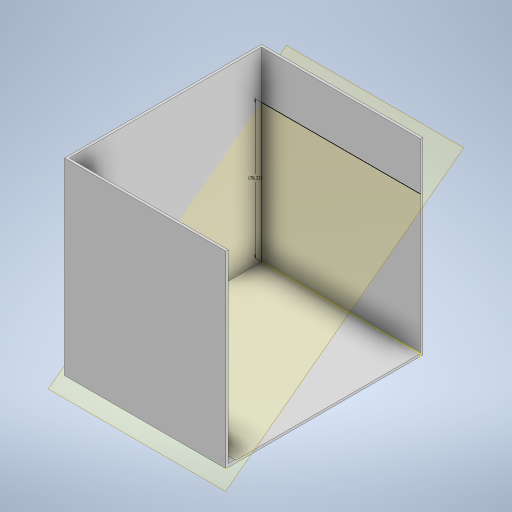
# Autodesk Inventor part: fullsembly
Saved by Autodesk Inventor 2024 (Build 280153000, 153)
## iProperties
Created: 2026-03-21
Part Number: fullsembly
Material: Generic
Document SubType Name: Modeling
Designer: schar
Density: 1 g/cm^3
Appearance: Default
Author: schar
Autodesk Inventor part; units mm, degrees
ref_plane "YZ Plane" through (0, 0, 0) normal (1, 0, 0) x (0, 1, 0)
ref_plane "XZ Plane" through (0, 0, 0) normal (0, 1, 0) x (-1, 0, 0)
ref_plane "XY Plane" through (0, 0, 0) normal (0, 0, 1) x (1, 0, 0)
sketch "Sketch1" plane through (0, 0, 0) normal (0, 1, 0) x (-1, 0, 0)
  line L0 (0, 0) -> (208, 0)
  line L1 (208, 0) -> (208, -254)
  line L2 (208, -254) -> (0, -254)
  line L3 (0, -254) -> (0, 0)
  dimension "d0" = 208
  dimension "d1" = 254
  constraints: 8 end point, 2 parallel, 1 horizontal, 1 perpendicular
  measures "d0" distance of L1.end L2.end
  measures "d1" distance of L0.end L1.end
extrude "Extrusion1" add sketch "Sketch1" along normal blind 3
sketch "Sketch2" plane through (0, 3, 0) normal (0, 1, 0) x (1, 0, 0)
  line L0 (0, 0) -> (0, 254) projected
  line L1 (-208, 254) -> (-208, 0) projected
  line L2 (0, 0) -> (-208, 0)
  line L3 (-208, 0) -> (-208, 3)
  line L4 (-208, 3) -> (0, 3)
  line L5 (0, 3) -> (0, 0)
  line L6 (0, 254) -> (-208, 254)
  line L7 (-208, 254) -> (-208, 251)
  line L8 (-208, 251) -> (0, 251)
  line L9 (0, 251) -> (0, 254)
  line L10 (-208, 3) -> (-205, 3)
  line L11 (-205, 3) -> (-205, 251)
  line L12 (-205, 251) -> (-208, 251)
  line L13 (-208, 251) -> (-208, 3)
  point P0 (-208, 0)
  point P1 (-205, 3)
  dimension "d4" = 3
  dimension "d5" = 3
  dimension "d6" = 3
  constraints: 24 end point, 6 parallel, 3 horizontal, 3 perpendicular, 3 point on line
  measures "d4" distance of L2.end L3.end
  measures "d5" distance of L7.end L6.end
  measures "d6" distance of L12.end L11.end
extrude "Extrusion2" add sketch "Sketch2" along normal blind 240 contours L2 L1 L4 L0 | L8 L1 L6 L0 | L4 L1 L8 L11
sketch "Sketch3" plane through (0, 0, 0) normal (1, 0, 0) x (0, 0, -1)
  point P0 (0, 0)
sketch "Sketch4" plane through (-205, 3, -3) normal (1, 0, 0) x (0, 0, -1)
  line L0 (0, 0) -> (1.4142, 0)
  line L1 (1.4142, 0) -> (1.4142, 1.4142)
  line L2 (1.4142, 1.4142) -> (0, 1.4142)
  line L3 (0, 1.4142) -> (0, 0)
  line L4 (0, 1.4142) -> (1.4142, 0)
  point P0 (-3, -3)
  dimension "d10" = 1.4142
  dimension "d11" = 1.4142
  constraints: 10 end point, 2 parallel, 1 horizontal, 1 perpendicular
  measures "d10" distance of L2.end L1.end
  measures "d11" distance of L1.end L0.end
extrude "Extrusion3" add sketch "Sketch4" along normal up to surface (205 mm away) contours L3 L4 L0
sketch "Sketch5" plane through (-205, 3, -251) normal (1, 0, 0) x (0, 0, -1)
  line L0 (-248, 1.4142) -> (-248, 240) projected
  line L1 (0, 0) -> (-246.5858, 0) projected
  line L2 (-248, 1.4142) -> (-238, 1.4142)
  line L3 (-238, 1.4142) -> (-238, 0)
  line L4 (-238, 0) -> (-248, 0)
  line L5 (-248, 0) -> (-248, 1.4142)
  point P0 (-251, -3)
  dimension "d14" = 10
  constraints: 8 end point, 2 parallel, 1 horizontal, 1 perpendicular, 1 point on line
  measures "d14" distance of L3.end L4.end
extrude "Extrusion4" add sketch "Sketch5" along normal up to surface (205 mm away)
sketch "Sketch6" plane through (0, 0, 0) normal (1, 0, 0) x (0, 0, -1)
  line L0 (13, 4.4142) -> (13, 3) projected
  line L1 (13, 3) -> (11.5858, 4.4142)
  line L2 (3, 4.4142) -> (13, 4.4142) projected
  line L3 (13, 4.4142) -> (11.5858, 4.4142)
  line L4 (13, 4.4142) -> (13, 3)
  point P0 (0, 0)
  dimension "d17" = 2
  constraints: 6 end point, 1 horizontal, 1 perpendicular, 1 point on line
  measures "d17" distance of L0.end L1.end
extrude "Extrusion5" cut sketch "Sketch6" against normal up to surface (205 mm away)
sketch "Sketch8" plane through (-205, 3, -251) normal (0, 0, 1) x (1, 0, 0)
  line L0 (205, 0) -> (0, 0) projected
  line L1 (-3, -3) -> (-3, 240) projected
  line L2 (0, 0) -> (0, 178.333)
  line L3 (0, 178.333) -> (205, 178.333)
  point P0 (205, -3)
  dimension "d25" = 178.333
  constraints: 4 end point, 1 horizontal, 1 parallel
  measures "d25" distance of L0.end L2.end
ref_plane "Work Plane1" through (-154.5, 3, -13) normal (0, 0.8002695, 0.5996406) x (1, 0, 0)
body "Solid1"
